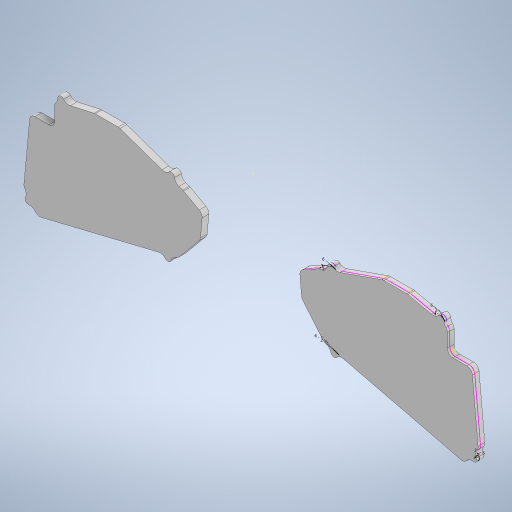
# Autodesk Inventor part: Деталь1
Saved by Autodesk Inventor 2024 (Build 280153000, 153)
## iProperties
Created: 2024-03-12
Part Number: Деталь1
Material: Типовые
Document SubType Name: Modeling
Designer: cepmi
Density: 1 g/cm^3
Appearance: По умолчанию
Autodesk Inventor part; units mm, degrees
ref_plane "YZ Plane" through (0, 0, 0) normal (1, 0, 0) x (0, 1, 0)
ref_plane "XZ Plane" through (0, 0, 0) normal (0, 1, 0) x (-1, 0, 0)
ref_plane "XY Plane" through (0, 0, 0) normal (0, 0, 1) x (1, 0, 0)
sketch "Эскиз2" plane through (0, 0, 0) normal (0, 0, 1) x (1, 0, 0)
  line L0 (198.9301, -55.8589) -> (204.052, -108.9276) projected
  line L1 (203.1202, -112.3468) -> (193.8602, -125.0922) projected
  line L2 (200.3335, -112.7798) -> (193.4165, -122.3003) projected
  arc A0 (200.3335, -112.7798) -> (201.2672, -109.3809) centre (196.2884, -109.8409) ccw projected
  line L3 (196.5134, -57.9292) -> (201.2672, -109.3809) projected
  arc A1 (203.1202, -112.3468) -> (204.052, -108.9276) centre (199.0752, -109.4079) ccw projected
  line L4 (181.4939, -51.3392) -> (193.9533, -51.3392) projected
  line L5 (179.4939, -53.3892) -> (191.5346, -53.3892) projected
  arc A2 (196.5134, -57.9292) -> (191.5346, -53.3892) centre (191.5346, -58.3892) ccw projected
  arc A3 (198.9301, -55.8589) -> (193.9533, -51.3392) centre (193.9533, -56.3392) ccw projected
  line L6 (64.659, -95.868) -> (46.5166, -74.0116) projected
  arc A4 (64.659, -95.868) -> (67.3256, -97.5331) centre (68.5062, -92.6745) ccw projected
  line L7 (60.3847, -86.3618) -> (48.3347, -71.8449) projected
  arc A5 (62.4853, -88.8923) -> (60.3847, -86.3618) centre (62.3109, -86.8999) ccw projected
  arc A6 (66.476, -93.7) -> (69.1455, -95.3658) centre (70.3233, -90.5065) ccw projected
  line L8 (66.476, -93.7) -> (62.4853, -88.8923) projected
  line L9 (119.3461, -22.1392) -> (139.9451, -22.1392) projected
  line L10 (141.0297, -22.2583) -> (172.5786, -29.2691) projected
  arc A7 (141.0297, -22.2583) -> (139.9451, -22.1392) centre (139.9451, -27.1392) ccw projected
  line L11 (121.3412, -24.1392) -> (137.9451, -24.1392) projected
  line L12 (139.0297, -24.2583) -> (141.5157, -24.8107) projected
  line L13 (145.0439, -25.5947) -> (170.5786, -31.2691) projected
  arc A8 (141.5157, -24.8107) -> (145.0439, -25.5947) centre (143.0939, -26.0392) ccw projected
  arc A9 (139.0297, -24.2583) -> (137.9451, -24.1392) centre (137.9451, -29.1392) ccw projected
  arc A10 (121.3412, -24.1392) -> (119.6939, -24.4183) centre (121.3412, -29.1392) ccw projected
  line L14 (61.3199, -42.212) -> (117.6898, -22.4215) projected
  arc A11 (119.3461, -22.1392) -> (117.6898, -22.4215) centre (119.3461, -27.1392) ccw projected
  arc A12 (61.3199, -42.212) -> (60.555, -42.555) centre (62.9762, -46.9297) ccw projected
  line L15 (63.4914, -44.0293) -> (119.6939, -24.4183) projected
  arc A13 (57.0981, -47.4855) -> (58.954, -46.4584) centre (58.8471, -48.4555) ccw projected
  line L16 (58.954, -46.4584) -> (62.7175, -44.3755) projected
  arc A14 (63.4914, -44.0293) -> (62.7175, -44.3755) centre (65.1386, -48.7501) ccw projected
  line L17 (176.4939, -34.1501) -> (176.4939, -46.3392) projected
  arc A15 (176.4939, -46.3392) -> (181.4939, -51.3392) centre (181.4939, -46.3392) ccw projected
  arc A16 (174.4939, -47.1392) -> (175.2292, -50.9991) centre (174.4939, -49.1392) ccw projected
  line L18 (174.4939, -36.1501) -> (174.4939, -47.1392) projected
  arc A17 (176.4939, -34.1501) -> (172.5786, -29.2691) centre (171.4939, -34.1501) ccw projected
  arc A18 (174.4939, -36.1501) -> (170.5786, -31.2691) centre (169.4939, -36.1501) ccw projected
  arc A19 (175.2292, -50.9991) -> (179.4939, -53.3892) centre (179.4939, -48.3892) ccw projected
  arc A20 (188.1936, -124.2207) -> (193.4165, -122.3003) centre (189.3714, -119.3614) ccw projected
  arc A21 (179.2918, -122.0631) -> (176.1952, -121.3125) centre (178.0283, -120.5127) ccw projected
  arc A22 (188.6344, -127.0119) -> (193.8602, -125.0922) centre (189.8151, -122.1533) ccw projected
  line L19 (188.1936, -124.2207) -> (179.2918, -122.0631) projected
  line L20 (45.3829, -71.2539) -> (43.9719, -55.1267) projected
  line L21 (46.5317, -50.3163) -> (60.555, -42.555) projected
  arc A23 (45.3829, -71.2539) -> (46.5166, -74.0116) centre (50.3639, -70.8181) ccw projected
  arc A24 (47.201, -69.0872) -> (48.3347, -71.8449) centre (52.1819, -68.6514) ccw projected
  line L22 (47.201, -69.0872) -> (46.1386, -56.9448) projected
  arc A25 (48.6984, -52.1343) -> (46.1386, -56.9448) centre (51.1196, -56.509) ccw projected
  line L23 (48.6984, -52.1343) -> (57.0981, -47.4855) projected
  arc A26 (46.5317, -50.3163) -> (43.9719, -55.1267) centre (48.9529, -54.691) ccw projected
  line L24 (188.6344, -127.0119) -> (67.3256, -97.5331) projected
  line L25 (176.1952, -121.3125) -> (69.1455, -95.3658) projected
  circle A27 centre (120.4939, -58.1392) radius 2 projected
  circle A28 centre (115.9939, -92.6392) radius 2 projected
  circle A29 centre (200.1083, -119.8951) radius 3
  line L26 (200.1083, -119.8951) -> (191.5299, -113.6625)
  circle A30 centre (71.6965, -36.4493) radius 3
  circle A31 centre (74.6787, -101.3781) radius 3
  circle A32 centre (170.6229, -26.7857) radius 3
  line L27 (170.6229, -26.7857) -> (168.2088, -37.649)
  line L28 (71.6965, -36.4493) -> (75.22, -46.4854)
  line L29 (74.6787, -101.3781) -> (78.1642, -87.0347)
  point P0 (0, 0)
  point P1 (198.4902, -118.7195)
  point P2 (65.858, -96.9156)
  point P3 (60.9302, -42.3675)
  point P4 (199.8046, -116.9105)
  point P5 (197.1759, -120.5285)
  point P6 (72.9781, -98.9067)
  point P7 (77.3238, -99.9627)
  point P8 (172.3718, -29.2232)
  point P9 (168.0062, -28.253)
  point P10 (74.4688, -37.5957)
  point P11 (70.2492, -39.0771)
  dimension "d4" = 6
  dimension "d5" = 2
  dimension "d6" = 6
  dimension "d7" = 6
  dimension "d8" = 6
  dimension "d9" = 2
  dimension "d12" = 2
  dimension "d13" = 2
  constraints: 8 end point, 4 centre point, 4 perpendicular, 2 point on circle, 1 midpoint, 1 point on line
  measures "d4" diameter of A29
  measures "d5" distance from line of L1 L26.start
  measures "d6" diameter of A30
  measures "d7" diameter of A31
  measures "d8" diameter of A32
  measures "d9" distance from line of L27.start L10
  measures "d12" distance from line of L14 L28.start
  measures "d13" distance from line of L24 L29.start
extrude "Выдавливание1" add sketch "Эскиз2" along normal blind 2 contours L0 A1 L1 A29 L26 L2 A0 L3 A2 L5 A19 A16 L18 A18 L13 L27 A32 L10 A17 L17 A15 L4 A3 | L1 L26 A29 | L1 A29 L26 | A29 L1 A22 L24 A31 L29 L25 A21 L19 A20 L2 L26 | L2 A20 L19 A21 L25 A6 L8 A5 L7 A24 L22 A25 L23 A13 L16 A14 L15 A10 L11 A9 L12 A8 L13 A18 L18 A16 A19 L5 A2 L3 A0 | A32 L27 L10 | L27 A32 L10 | L27 L13 A8 L12 A9 L11 A10 L15 L28 A30 L14 A11 L9 A7 L10 A32 | L24 L29 A31 | L24 A31 L29 | A31 L24 A4 L6 A23 L20 A26 L21 A12 L14 A30 L28 L15 A14 L16 A13 L23 A25 L22 A24 L7 A5 L8 A6 L25 L29 | A30 L28 L14 | L28 A30 L14 | A27 | A28
extrude "Выдавливание2" add sketch "Эскиз2" against normal blind 4 contours L0 A1 L1 A29 L26 L2 A0 L3 A2 L5 A19 A16 L18 A18 L13 L27 A32 L10 A17 L17 A15 L4 A3 | L1 L26 A29 | L1 A29 L26 | A29 L1 A22 L24 A31 L29 L25 A21 L19 A20 L2 L26 | A32 L27 L10 | L27 A32 L10 | L27 L13 A8 L12 A9 L11 A10 L15 L28 A30 L14 A11 L9 A7 L10 A32 | L24 L29 A31 | L24 A31 L29 | A31 L24 A4 L6 A23 L20 A26 L21 A12 L14 A30 L28 L15 A14 L16 A13 L23 A25 L22 A24 L7 A5 L8 A6 L25 L29 | A30 L28 L14 | L28 A30 L14 | A27 | A28
extrude "Выдавливание3" add sketch "Эскиз2" against normal blind 4 contours A29 L1 | A32 L27 L10 | L10 A32 | L27 A32 L10 | A31 L24 | A30 L28 L14 | L14 A30 | L28 A30 L14
extrude "Выдавливание4" add sketch "Эскиз2" along normal blind 2 contours A29 L1 | L1 L26 A29 | L1 A29 L26 | L10 A32 | A31 L24 | L24 L29 A31 | L24 A31 L29 | L14 A30
fillet "Сопряжение1" radius 6 16 edges at (72.9781, -98.9067, -2) (72.9781, -98.9067, 1) (70.2492, -39.0771, 1) (70.2492, -39.0771, -2) (172.3718, -29.2232, -2) (172.3718, -29.2232, 1) (77.3238, -99.9627, 1) (77.3238, -99.9627, -2) (74.4688, -37.5957, -2) (74.4688, -37.5957, 1) (199.8046, -116.9105, 1) (199.8046, -116.9105, -2) (168.0062, -28.253, 1) (168.0062, -28.253, -2) (197.1759, -120.5285, -2) (197.1759, -120.5285, 1)
mirror "Зеркальное отражение1" about plane through (0, 0, 0) normal (1, 0, 0) of "Выдавливание2", "Выдавливание3", "Выдавливание4", "Сопряжение1", "Выдавливание1"
